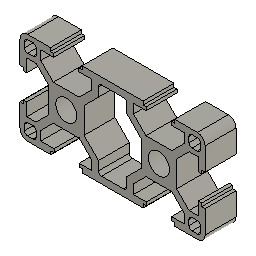
_30mm x 60mm Profile v4.02e2be94-0d6a-477b-a073-dc361f5778b3 (Autodesk Fusion 360 design; units mm, degrees)
Autodesk Fusion 360 part; units mm, degrees
sketch "Sketch1" plane through (0, 0, 0) normal (0, 1, 0) x (1, 0, 0)
  circle A0 centre (0, 0) radius 3.4
  circle A1 centre (30, 0) radius 3.4244
  line L0 (-12.8, 8.25) -> (-9.8056, 8.25)
  line L1 (-12.8, -8.25) -> (-9.8056, -8.25)
  line L2 (39.8056, -8.25) -> (42.8, -8.25)
  line L3 (39.8056, 8.25) -> (42.8, 8.25)
  line L4 (38.25, -12.8) -> (38.25, -9.8056)
  line L5 (38.25, 9.8056) -> (38.25, 12.8)
  line L6 (-8.25, -12.8) -> (-8.25, -9.8056)
  line L7 (-8.25, 9.8056) -> (-8.25, 12.8)
  line L8 (4.1944, 5.75) -> (-4.1944, 5.75)
  line L9 (-5.75, 4.1944) -> (-5.75, -4.1944)
  line L10 (-4.1944, -5.75) -> (4.1944, -5.75)
  line L11 (5.75, -4.1944) -> (5.75, 4.1944)
  line L12 (34.1944, 5.75) -> (25.8056, 5.75)
  line L13 (24.25, 4.1944) -> (24.25, -4.1944)
  line L14 (25.8056, -5.75) -> (34.1944, -5.75)
  line L15 (35.75, -4.1944) -> (35.75, 4.1944)
  line L16 (35.75, 5.75) -> (24.25, -5.75) construction
  line L17 (24.25, 5.75) -> (35.75, -5.75) construction
  line L18 (-8.25, -9.8056) -> (-4.1944, -5.75)
  line L19 (-9.8056, -8.25) -> (-5.75, -4.1944)
  line L20 (-9.8056, 8.25) -> (-5.75, 4.1944)
  line L21 (-8.25, 9.8056) -> (-4.1944, 5.75)
  line L22 (4.1944, 5.75) -> (8.25, 9.8056)
  line L23 (5.75, 4.1944) -> (9.515, 7.9594)
  line L24 (5.75, -4.1944) -> (10.45, -8.8944)
  line L25 (4.1944, -5.75) -> (8.25, -9.8056)
  line L26 (5.75, 5.75) -> (-0.7778, -0.7778) construction
  line L27 (-2.4042, -2.4042) -> (-5.75, -5.75) construction
  line L28 (-8.25, 8.25) -> (-2.4042, 2.4042) construction
  line L29 (0, 0) -> (15, -15) construction
  line L30 (15, 15) -> (5.75, 5.75) construction
  line L31 (2.4042, 2.4042) -> (-13.2071, -13.2071) construction
  line L32 (8.25, 9.8056) -> (8.25, 12.8)
  line L33 (8.25, -12.8) -> (8.25, -9.8056)
  line L34 (9.515, 7.9594) -> (10.45, 8.8944)
  line L35 (10.45, -11.8) -> (10.45, -8.8944)
  line L36 (10.45, 8.8944) -> (10.45, 11.8)
  line L37 (21.75, 9.8056) -> (21.75, 12.8)
  line L38 (21.3592, -7.0851) -> (19.55, -8.8944)
  line L39 (21.75, -12.8) -> (21.75, -9.8056)
  line L40 (15, -15) -> (24.25, -5.75) construction
  line L41 (27.5786, -2.4214) -> (38.25, 8.25) construction
  line L42 (21.3592, -7.0851) -> (24.25, -4.1944)
  line L43 (25.8056, -5.75) -> (21.75, -9.8056)
  line L44 (19.55, 8.8944) -> (24.25, 4.1944)
  line L45 (21.75, 9.8056) -> (25.8056, 5.75)
  line L46 (19.55, -11.8) -> (19.55, -8.8944)
  line L47 (19.55, 8.8944) -> (19.55, 11.8)
  line L48 (34.1944, 5.75) -> (38.25, 9.8056)
  line L49 (39.8056, 8.25) -> (35.75, 4.1944)
  line L50 (35.75, -4.1944) -> (39.8056, -8.25)
  line L51 (34.1944, -5.75) -> (38.25, -9.8056)
  line L52 (32.4214, -2.4214) -> (15, 15) construction
  line L53 (42.8, -4.1) -> (43.9, -4.1)
  line L54 (42.8, 4.1) -> (43.9, 4.1)
  line L55 (43.9, 5.1) -> (45, 5.1)
  line L56 (25.9, -12.8) -> (25.9, -13.9)
  line L57 (24.9, -15) -> (24.9, -13.9)
  line L58 (34.1, -13.9) -> (34.1, -12.8)
  line L59 (35.1, -15) -> (35.1, -13.9)
  line L60 (4.1, -13.9) -> (4.1, -12.8)
  line L61 (5.1, -15) -> (5.1, -13.9)
  line L62 (-4.1, -13.9) -> (-4.1, -12.8)
  line L63 (-5.1, -15) -> (-5.1, -13.9)
  line L64 (-12.8, -4.1) -> (-13.9, -4.1)
  line L65 (-15, -5.1) -> (-13.9, -5.1)
  line L66 (-13.9, 4.1) -> (-12.8, 4.1)
  line L67 (-13.9, 5.1) -> (-15, 5.1)
  line L68 (-3.9717, 12.8) -> (-3.9717, 13.9)
  line L69 (-4.9717, 13.9) -> (-4.9717, 15)
  line L70 (4.1673, 12.8) -> (4.1673, 13.9)
  line L71 (5.1673, 13.9) -> (5.1673, 15)
  line L72 (24.9, 13.9) -> (24.9, 15)
  line L73 (25.9, 12.8) -> (25.9, 13.9)
  line L74 (34.1, 12.8) -> (34.1, 13.9)
  line L75 (35.1, 13.9) -> (35.1, 15)
  line L76 (34.1, -12.8) -> (38.25, -12.8)
  line L77 (35.1, -15) -> (42.5, -15)
  line L78 (43.9, -5.1) -> (45, -5.1)
  line L79 (45, -12.5) -> (45, -5.1)
  line L80 (45, 5.1) -> (45, 12.5)
  line L81 (42.8, -8.25) -> (42.8, -4.1)
  line L82 (42.8, 4.1) -> (42.8, 8.25)
  line L83 (34.1, 12.8) -> (38.25, 12.8)
  line L84 (35.1, 15) -> (42.5, 15)
  line L85 (-12.5, 15) -> (-4.9717, 15)
  line L86 (5.1673, 15) -> (24.9, 15)
  line L87 (-8.25, 12.8) -> (-3.9717, 12.8)
  line L88 (-12.8, -8.25) -> (-12.8, -4.1)
  line L89 (-12.8, 4.1) -> (-12.8, 8.25)
  line L90 (-15, -12.5) -> (-15, -5.1)
  line L91 (-15, 5.1) -> (-15, 12.5)
  line L92 (-5.75, 5.75) -> (-2.4042, 2.4042) construction
  line L93 (0, 0) -> (2.4042, -2.4042) construction
  line L94 (-12.5, -15) -> (-5.1, -15)
  line L95 (5.1, -15) -> (24.9, -15)
  line L96 (-8.25, -12.8) -> (-4.1, -12.8)
  line L97 (4.1, -12.8) -> (8.25, -12.8)
  line L98 (11.45, -12.8) -> (18.55, -12.8)
  line L99 (21.75, -12.8) -> (25.9, -12.8)
  line L100 (21.75, 12.8) -> (25.9, 12.8)
  line L101 (4.1673, 12.8) -> (8.25, 12.8)
  line L102 (11.45, 12.8) -> (18.55, 12.8)
  line L103 (-13.9, -5.1) -> (-13.9, -4.1)
  line L104 (-13.9, 4.1) -> (-13.9, 5.1)
  line L105 (-5.1, -13.9) -> (-4.1, -13.9)
  line L106 (4.1, -13.9) -> (5.1, -13.9)
  line L107 (24.9, -13.9) -> (25.9, -13.9)
  line L108 (34.1, -13.9) -> (35.1, -13.9)
  line L109 (43.9, -5.1) -> (43.9, -4.1)
  line L110 (43.9, 4.1) -> (43.9, 5.1)
  line L111 (34.1, 13.9) -> (35.1, 13.9)
  line L112 (24.9, 13.9) -> (25.9, 13.9)
  line L113 (-4.9717, 13.9) -> (-3.9717, 13.9)
  line L114 (4.1673, 13.9) -> (5.1673, 13.9)
  line L115 (-12.5, -9.75) -> (-10.75, -9.75)
  line L116 (-9.75, -10.75) -> (-9.75, -12.5)
  line L117 (-10.75, -13.5) -> (-12.5, -13.5)
  line L118 (-13.5, -12.5) -> (-13.5, -10.75)
  arc A2 (-10.75, -13.5) -> (-9.75, -12.5) centre (-10.75, -12.5) ccw
  arc A3 (-13.5, -12.5) -> (-12.5, -13.5) centre (-12.5, -12.5) ccw
  arc A4 (-12.5, -9.75) -> (-13.5, -10.75) centre (-12.5, -10.75) ccw
  arc A5 (-9.75, -10.75) -> (-10.75, -9.75) centre (-10.75, -10.75) ccw
  arc A6 (-15, -12.5) -> (-12.5, -15) centre (-12.5, -12.5) ccw
  line L119 (-12.5, 13.5) -> (-10.75, 13.5)
  line L120 (-9.75, 12.5) -> (-9.75, 10.75)
  line L121 (-10.75, 9.75) -> (-12.5, 9.75)
  line L122 (-13.5, 10.75) -> (-13.5, 12.5)
  arc A7 (-10.75, 9.75) -> (-9.75, 10.75) centre (-10.75, 10.75) ccw
  arc A8 (-13.5, 10.75) -> (-12.5, 9.75) centre (-12.5, 10.75) ccw
  arc A9 (-12.5, 13.5) -> (-13.5, 12.5) centre (-12.5, 12.5) ccw
  arc A10 (-9.75, 12.5) -> (-10.75, 13.5) centre (-10.75, 12.5) ccw
  arc A11 (-12.5, 15) -> (-15, 12.5) centre (-12.5, 12.5) ccw
  line L123 (40.75, -9.75) -> (42.5, -9.75)
  line L124 (43.5, -10.75) -> (43.5, -12.5)
  line L125 (42.5, -13.5) -> (40.75, -13.5)
  line L126 (39.75, -12.5) -> (39.75, -10.75)
  arc A12 (42.5, -13.5) -> (43.5, -12.5) centre (42.5, -12.5) ccw
  arc A13 (39.75, -12.5) -> (40.75, -13.5) centre (40.75, -12.5) ccw
  arc A14 (40.75, -9.75) -> (39.75, -10.75) centre (40.75, -10.75) ccw
  arc A15 (43.5, -10.75) -> (42.5, -9.75) centre (42.5, -10.75) ccw
  arc A16 (42.5, -15) -> (45, -12.5) centre (42.5, -12.5) ccw
  line L127 (40.75, 13.5) -> (42.5, 13.5)
  line L128 (43.5, 12.5) -> (43.5, 10.75)
  line L129 (42.5, 9.75) -> (40.75, 9.75)
  line L130 (39.75, 10.75) -> (39.75, 12.5)
  arc A17 (42.5, 9.75) -> (43.5, 10.75) centre (42.5, 10.75) ccw
  arc A18 (43.5, 12.5) -> (42.5, 13.5) centre (42.5, 12.5) ccw
  arc A19 (40.75, 13.5) -> (39.75, 12.5) centre (40.75, 12.5) ccw
  arc A20 (39.75, 10.75) -> (40.75, 9.75) centre (40.75, 10.75) ccw
  arc A21 (45, 12.5) -> (42.5, 15) centre (42.5, 12.5) ccw
  arc A22 (10.45, -11.8) -> (11.45, -12.8) centre (11.45, -11.8) ccw
  arc A23 (18.55, -12.8) -> (19.55, -11.8) centre (18.55, -11.8) ccw
  arc A24 (19.55, 11.8) -> (18.55, 12.8) centre (18.55, 11.8) ccw
  arc A25 (11.45, 12.8) -> (10.45, 11.8) centre (11.45, 11.8) ccw
  point P0 (30, 0)
  point P1 (-13.5, -9.75)
  point P2 (-9.75, -13.5)
  point P3 (-13.5, -13.5)
  point P4 (-9.75, 13.5)
  point P5 (-9.75, 9.75)
  point P6 (-13.5, 9.75)
  point P7 (43.5, -9.75)
  point P8 (43.5, -13.5)
  point P9 (39.75, -13.5)
  point P10 (39.75, 13.5)
  point P11 (43.5, 9.75)
  point P12 (39.75, 9.75)
  dimension "d1" = 6.8
  dimension "d2" = 15
  dimension "d3" = 15
  dimension "d4" = 15
  dimension "d5" = 45
  dimension "d6" = 30
  dimension "d7" = 2.2
  dimension "d8" = 2.2
  dimension "d9" = 2.2
  dimension "d10" = 2.2
  dimension "d11" = 8.25
  dimension "d12" = 8.25
  dimension "d13" = 8.25
  dimension "d14" = 8.25
  dimension "d15" = 8.25
  dimension "d18" = 2.2
  dimension "d19" = 1.1
  dimension "d20" = 1.1
  dimension "d21" = 1.1
  dimension "d22" = 1.1
  dimension "d23" = 1.1
  dimension "d24" = 1.1
  dimension "d25" = 1.1
  dimension "d26" = 1.1
  dimension "d28" = 11.5
  dimension "d29" = 11.5
  dimension "d30" = 11.5
  dimension "d31" = 4.1
  dimension "d32" = 4.1
  dimension "d34" = 1
  dimension "d35" = 4.1
  dimension "d36" = 1
  dimension "d37" = 4.1
  dimension "d38" = 1
  dimension "d39" = 4.1
  dimension "d40" = 4.1
  dimension "d42" = 1
  dimension "d43" = 1
  dimension "d44" = 1
  dimension "d45" = 4.1
  dimension "d46" = 1
  dimension "d47" = 4.1
  dimension "d48" = 1
  dimension "d49" = 4.1
  dimension "d50" = 4.1
  dimension "d51" = 1
  dimension "d52" = 1
  dimension "d53" = 1.1
  dimension "d55" = 1.1
  dimension "d56" = 1.1
  dimension "d57" = 3.75
  dimension "d58" = 3.75
  dimension "d59" = 1.5
  dimension "d60" = 1.5
  dimension "d61" = 1
  dimension "d62" = 2.5
  dimension "d63" = 3.75
  dimension "d64" = 3.75
  dimension "d65" = 1.5
  dimension "d66" = 1.5
  dimension "d67" = 1
  dimension "d68" = 2.5
  dimension "d69" = 1
  dimension "d70" = 1
  dimension "d71" = 3.75
  dimension "d72" = 3.75
  dimension "d73" = 1.5
  dimension "d74" = 1.5
  dimension "d75" = 1
  dimension "d76" = 2.5
  dimension "d77" = 3.75
  dimension "d78" = 3.75
  dimension "d79" = 1.5
  dimension "d80" = 1.5
  dimension "d81" = 1
  dimension "d82" = 2.5
  dimension "d83" = 1
  constraint coincident A0.centre L29.start
  constraint horizontal L94
  constraint parallel L85 L94
  constraint perpendicular L85 L90
  constraint perpendicular L79 L85
  constraint horizontal A0.centre P0
  constraint parallel L85 L87
  constraint parallel L87 L96
  constraint perpendicular L81 L94
  constraint parallel L81 L88
  constraint perpendicular L6 L85
  constraint perpendicular L33 L87
  constraint perpendicular L39 L87
  constraint perpendicular L4 L85
  constraint coincident L33.start L96
  constraint coincident L39.start L96
  constraint coincident L37.end L87
  constraint coincident L32.end L87
  constraint perpendicular L1 L79
  constraint coincident L28.start L6
  constraint collinear L0 L3
  constraint collinear L1 L2
  constraint coincident L41.end L4
  constraint collinear L4 L5
  constraint collinear L6 L7
  constraint perpendicular L35 L85
  constraint perpendicular L20 L30
  constraint parallel L20 L21
  constraint perpendicular L40 L45
  constraint perpendicular L45 L49
  constraint perpendicular L42 L45
  constraint perpendicular L18 L21
  constraint perpendicular L19 L21
  constraint horizontal L8
  constraint perpendicular L8 L9
  constraint parallel L8 L10
  constraint parallel L9 L11
  constraint coincident A0.centre L26
  constraint coincident A0.centre L92
  constraint horizontal L12
  constraint perpendicular L12 L13
  constraint parallel L12 L14
  constraint parallel L13 L15
  constraint coincident L16.start L40
  constraint coincident L16 P0
  constraint coincident L17 P0
  constraint coincident P0 A1.centre
  constraint coincident L26.end L30
  constraint coincident A0 L27.start
  constraint collinear L26 L27
  constraint collinear L28 L29
  constraint coincident A0 L28.end
  constraint coincident A0 L31.start
  constraint collinear L30 L31
  constraint collinear L32 L33
  constraint coincident L34.end L35
  constraint parallel L23 L34
  constraint collinear L35 L36
  constraint coincident A0 L93.end
  constraint coincident L44.start L46
  constraint coincident L37.start L39
  constraint collinear L37 L39
  constraint parallel L38 L42
  constraint coincident A1 L41.start
  constraint collinear L40 L41
  constraint coincident L14.start L49
  constraint collinear L43 L49
  constraint collinear L46 L47
  constraint coincident A1 L52.start
  constraint perpendicular L53 L79
  constraint perpendicular L54 L79
  constraint perpendicular L55 L79
  constraint perpendicular L56 L94
  constraint perpendicular L57 L96
  constraint perpendicular L58 L96
  constraint perpendicular L59 L96
  constraint perpendicular L60 L96
  constraint perpendicular L61 L96
  constraint perpendicular L62 L96
  constraint perpendicular L63 L96
  constraint perpendicular L64 L90
  constraint perpendicular L65 L90
  constraint perpendicular L66 L88
  constraint perpendicular L67 L90
  constraint perpendicular L68 L85
  constraint perpendicular L69 L85
  constraint perpendicular L70 L85
  constraint perpendicular L71 L85
  constraint perpendicular L72 L85
  constraint perpendicular L73 L85
  constraint perpendicular L74 L85
  constraint perpendicular L75 L85
  constraint coincident L54.start L81
  constraint coincident L55.end L79
  constraint coincident L58.end L96
  constraint collinear L76 L96
  constraint coincident L57.start L94
  constraint collinear L77 L94
  constraint coincident L29.end L94
  constraint perpendicular L78 L81
  constraint coincident L74.start L87
  constraint coincident L75.end L85
  constraint collinear L79 L80
  constraint collinear L81 L82
  constraint coincident L72.end L85
  constraint collinear L83 L87
  constraint collinear L84 L85
  constraint coincident L30.start L85
  constraint coincident L70.start L87
  constraint coincident L71.end L85
  constraint collinear L85 L86
  constraint collinear L87 L101
  constraint coincident L67.end L90
  constraint coincident L66.end L88
  constraint collinear L88 L89
  constraint collinear L90 L91
  constraint collinear L92 L93
  constraint coincident L60.end L96
  constraint coincident L61.start L94
  constraint collinear L94 L95
  constraint collinear L96 L97
  constraint collinear L97 L98
  constraint collinear L98 L99
  constraint collinear L100 L101
  constraint collinear L101 L102
  constraint perpendicular L67 L103
  constraint perpendicular L80 L113
  constraint perpendicular L55 L109
  constraint perpendicular L59 L105
  constraint coincident L66.start L103
  constraint collinear L103 L104
  constraint coincident L60.start L105
  constraint collinear L105 L107
  constraint collinear L105 L106
  constraint coincident L58.start L107
  constraint collinear L107 L108
  constraint collinear L109 L110
  constraint collinear L111 L113
  constraint coincident L72.start L113
  constraint collinear L112 L113
  constraint coincident L70.end L113
  constraint collinear L113 L114
  constraint horizontal L115
  constraint vertical L116
  constraint horizontal L117
  constraint vertical L118
  constraint coincident P2 L116
  constraint coincident P2 L117
  constraint tangent L116 A2
  constraint tangent L117 A2
  constraint coincident P3 L117
  constraint coincident P3 L118
  constraint tangent L117 A3
  constraint tangent L118 A3
  constraint equal A2 A3
  constraint coincident P1 L115
  constraint coincident P1 L118
  constraint tangent L115 A4
  constraint tangent L118 A4
  constraint equal A2 A4
  constraint tangent L115 A5
  constraint tangent L116 A5
  constraint equal A2 A5
  constraint coincident A3 L31.end
  constraint tangent L90 A6
  constraint tangent L94 A6
  constraint horizontal L119
  constraint vertical L120
  constraint horizontal L121
  constraint vertical L122
  constraint coincident P5 L120
  constraint coincident P5 L121
  constraint tangent L120 A7
  constraint tangent L121 A7
  constraint coincident P6 L121
  constraint coincident P6 L122
  constraint tangent L121 A8
  constraint tangent L122 A8
  constraint equal A7 A8
  constraint tangent L119 A9
  constraint tangent L122 A9
  constraint equal A7 A9
  constraint coincident P4 L119
  constraint coincident P4 L120
  constraint tangent L119 A10
  constraint tangent L120 A10
  constraint equal A7 A10
  constraint tangent L85 A11
  constraint tangent L91 A11
  constraint horizontal L123
  constraint vertical L124
  constraint horizontal L125
  constraint vertical L126
  constraint coincident P8 L124
  constraint coincident P8 L125
  constraint tangent L124 A12
  constraint tangent L125 A12
  constraint coincident P9 L125
  constraint coincident P9 L126
  constraint tangent L125 A13
  constraint tangent L126 A13
  constraint equal A12 A13
  constraint tangent L123 A14
  constraint tangent L126 A14
  constraint equal A12 A14
  constraint coincident P7 L123
  constraint coincident P7 L124
  constraint tangent L123 A15
  constraint tangent L124 A15
  constraint equal A12 A15
  constraint tangent L77 A16
  constraint tangent L79 A16
  constraint horizontal L127
  constraint vertical L128
  constraint horizontal L129
  constraint vertical L130
  constraint coincident P11 L128
  constraint coincident P11 L129
  constraint tangent L128 A17
  constraint tangent L129 A17
  constraint tangent L127 A18
  constraint tangent L128 A18
  constraint equal A17 A18
  constraint coincident P10 L127
  constraint coincident P10 L130
  constraint tangent L127 A19
  constraint tangent L130 A19
  constraint equal A17 A19
  constraint coincident P12 L129
  constraint coincident P12 L130
  constraint tangent L129 A20
  constraint tangent L130 A20
  constraint equal A17 A20
  constraint tangent L80 A21
  constraint tangent L84 A21
  constraint tangent L35 A22
  constraint tangent L98 A22
  constraint tangent L46 A23
  constraint tangent L98 A23
  constraint equal A22 A23
  constraint tangent L47 A24
  constraint tangent L102 A24
  constraint equal A22 A24
  constraint tangent L36 A25
  constraint tangent L102 A25
  constraint equal A22 A25
  measures "d1" diameter of A0
  measures "d2" distance of A0.centre L94
  measures "d3" distance of A0.centre L85
  measures "d4" distance of A0.centre L90
  measures "d5" distance of A0.centre L79
  measures "d6" horizontal distance of A0.centre A1.centre
  measures "d7" distance of L94 L96
  measures "d8" distance of L85 L87
  measures "d9" distance of L79 L81
  measures "d10" distance of L88 L90
  measures "d11" distance of A0.centre L33
  measures "d12" distance of A0.centre L6
  measures "d13" distance of P0 L39
  measures "d14" distance of P0 L4
  measures "d15" distance of A0.centre L1
  measures "d18" distance of L33 L35
  measures "d19" distance of P0 L44
  measures "d20" distance of P0 L45
  measures "d21" distance of P0 L49
  measures "d22" distance of P0 L42
  measures "d23" distance of L21 L28
  measures "d24" distance of L20 L28
  measures "d25" distance of A0.centre L18
  measures "d26" distance of A0.centre L19
  measures "d28" distance of L92.start L27.end
  measures "d29" distance of L16.end L17.end
  measures "d30" distance of L16.start L17.end
  measures "d31" distance of P0 L53
  measures "d32" distance of P0 L54
  measures "d34" distance of L54 L55
  measures "d35" distance of P0 L74
  measures "d36" distance of L74 L75
  measures "d37" distance of P0 L73
  measures "d38" distance of L72 L73
  measures "d39" distance of P0 L58
  measures "d40" distance of P0 L56
  measures "d42" distance of L56 L57
  measures "d43" distance of L58 L59
  measures "d44" distance of L53 L78
  measures "d45" distance of A0.centre L64
  measures "d46" distance of L64 L65
  measures "d47" distance of A0.centre L66
  measures "d48" distance of L66 L67
  measures "d49" distance of A0.centre L62
  measures "d50" distance of A0.centre L60
  measures "d51" distance of L60 L61
  measures "d52" distance of L62 L63
  measures "d53" distance of L95 L105
  measures "d55" distance of L79 L109
  measures "d56" distance of L90 L103
  measures "d57" distance of P2 P3
  measures "d58" distance of P1 P3
  measures "d59" distance of L90 L118
  measures "d60" distance of L94 L117
  measures "d61" radius of A2
  measures "d62" radius of A6
  measures "d63" distance of P5 P6
  measures "d64" distance of P4 P5
  measures "d65" distance of L91 L122
  measures "d66" distance of L85 L119
  measures "d67" radius of A7
  measures "d68" radius of A11
  measures "d69" distance of L68 L69
  measures "d70" distance of L70 L71
  measures "d71" distance of P8 P9
  measures "d72" distance of P7 P8
  measures "d73" distance of L79 L124
  measures "d74" distance of L77 L125
  measures "d75" radius of A12
  measures "d76" radius of A16
  measures "d77" distance of P11 P12
  measures "d78" distance of P10 P12
  measures "d79" distance of L80 L128
  measures "d80" distance of L84 L127
  measures "d81" radius of A17
  measures "d82" radius of A21
  measures "d83" radius of A22
extrude "Extrude1" add sketch "Sketch1" along normal blind 500 in component "Component"
extrude "Extrude2" cut 1 faces at (-0.0847, 500, 4.9635) along direction (0, -1, 0) blind 490 in component "Component"
component "Component" placed x (1, 0, 0) y (0, 1, 0) z (0, 0, 1) at (0, 0, 0)
